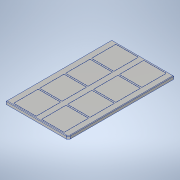
# Autodesk Inventor part: Assembly Plate
Saved by Autodesk Inventor 2022 (Build 260153000, 153)
## iProperties
Created: 2021-01-11
Part Number: Assembly Plate
Material: Aluminum 6061
Document SubType Name: Modeling
Designer: caleb
Density: 2.7 g/cm^3
Appearance: Aluminum - Flat
Author: caleb
Autodesk Inventor part; units mm, degrees
ref_plane "YZ Plane" through (0, 0, 0) normal (1, 0, 0) x (0, 1, 0)
ref_plane "XZ Plane" through (0, 0, 0) normal (0, 1, 0) x (-1, 0, 0)
ref_plane "XY Plane" through (0, 0, 0) normal (0, 0, 1) x (1, 0, 0)
sketch "Sketch1" plane through (0, 0, 0) normal (0, 1, 0) x (-1, 0, 0)
  line L0 (-63.5, 107.95) -> (63.5, 107.95)
  line L1 (63.5, 107.95) -> (63.5, -107.95)
  line L2 (63.5, -107.95) -> (-63.5, -107.95)
  line L3 (-63.5, -107.95) -> (-63.5, 107.95)
  line L4 (-63.5, 107.95) -> (63.5, -107.95) construction
  line L5 (63.5, 107.95) -> (-63.5, -107.95) construction
  point P0 (0, 0)
  dimension "d0" = 127
  dimension "d1" = 215.9
  constraints: 12 end point, 2 midpoint, 2 parallel, 1 horizontal, 1 perpendicular
  measures "d0" distance of L1.end L2.end
  measures "d1" distance of L0.end L1.end
extrude "Extrusion1" add sketch "Sketch1" along normal blind 6.35
sketch "Sketch8" plane through (0, 6.35, 0) normal (0, 1, 0) x (1, 0, 0)
  line L0 (-50.5, 104.45) -> (-6.5, 104.45)
  line L1 (-5.5, 103.45) -> (-5.5, 55.45)
  line L2 (-6.5, 54.45) -> (-50.5, 54.45)
  line L3 (-51.5, 55.45) -> (-51.5, 103.45)
  line L4 (63.5, 107.95) -> (-63.5, 107.95) projected
  line L5 (-63.5, -107.95) -> (63.5, -107.95) projected
  line L6 (-63.5, 107.95) -> (-63.5, -107.95) projected
  line L7 (63.5, -107.95) -> (63.5, 107.95) projected
  arc A0 (-51.5, 55.45) -> (-50.5, 54.45) centre (-50.5, 55.45) ccw
  arc A1 (-6.5, 54.45) -> (-5.5, 55.45) centre (-6.5, 55.45) ccw
  arc A2 (-5.5, 103.45) -> (-6.5, 104.45) centre (-6.5, 103.45) ccw
  arc A3 (-50.5, 104.45) -> (-51.5, 103.45) centre (-50.5, 103.45) ccw
  line L8 (-50.5, 51.45) -> (-6.5, 51.45)
  arc A4 (-50.5, 51.45) -> (-51.5, 50.45) centre (-50.5, 50.45) ccw
  arc A5 (-5.5, 50.45) -> (-6.5, 51.45) centre (-6.5, 50.45) ccw
  line L9 (-51.5, 2.45) -> (-51.5, 50.45)
  line L10 (-5.5, 50.45) -> (-5.5, 2.45)
  line L11 (-6.5, 1.45) -> (-50.5, 1.45)
  arc A6 (-6.5, 1.45) -> (-5.5, 2.45) centre (-6.5, 2.45) ccw
  arc A7 (-51.5, 2.45) -> (-50.5, 1.45) centre (-50.5, 2.45) ccw
  line L12 (-50.5, -1.55) -> (-6.5, -1.55)
  arc A8 (-50.5, -1.55) -> (-51.5, -2.55) centre (-50.5, -2.55) ccw
  arc A9 (-5.5, -2.55) -> (-6.5, -1.55) centre (-6.5, -2.55) ccw
  line L13 (-51.5, -50.55) -> (-51.5, -2.55)
  line L14 (-5.5, -2.55) -> (-5.5, -50.55)
  line L15 (-6.5, -51.55) -> (-50.5, -51.55)
  arc A10 (-6.5, -51.55) -> (-5.5, -50.55) centre (-6.5, -50.55) ccw
  arc A11 (-51.5, -50.55) -> (-50.5, -51.55) centre (-50.5, -50.55) ccw
  line L16 (-50.5, -54.55) -> (-6.5, -54.55)
  arc A12 (-50.5, -54.55) -> (-51.5, -55.55) centre (-50.5, -55.55) ccw
  arc A13 (-5.5, -55.55) -> (-6.5, -54.55) centre (-6.5, -55.55) ccw
  line L17 (-51.5, -103.55) -> (-51.5, -55.55)
  line L18 (-5.5, -55.55) -> (-5.5, -103.55)
  line L19 (-6.5, -104.55) -> (-50.5, -104.55)
  arc A14 (-6.5, -104.55) -> (-5.5, -103.55) centre (-6.5, -103.55) ccw
  arc A15 (-51.5, -103.55) -> (-50.5, -104.55) centre (-50.5, -103.55) ccw
  line L20 (6.5, 104.45) -> (50.5, 104.45)
  arc A16 (6.5, 104.45) -> (5.5, 103.45) centre (6.5, 103.45) ccw
  arc A17 (51.5, 103.45) -> (50.5, 104.45) centre (50.5, 103.45) ccw
  line L21 (5.5, 55.45) -> (5.5, 103.45)
  line L22 (51.5, 103.45) -> (51.5, 55.45)
  line L23 (50.5, 54.45) -> (6.5, 54.45)
  arc A18 (50.5, 54.45) -> (51.5, 55.45) centre (50.5, 55.45) ccw
  arc A19 (5.5, 55.45) -> (6.5, 54.45) centre (6.5, 55.45) ccw
  line L24 (6.5, 51.45) -> (50.5, 51.45)
  arc A20 (6.5, 51.45) -> (5.5, 50.45) centre (6.5, 50.45) ccw
  arc A21 (51.5, 50.45) -> (50.5, 51.45) centre (50.5, 50.45) ccw
  line L25 (5.5, 2.45) -> (5.5, 50.45)
  line L26 (51.5, 50.45) -> (51.5, 2.45)
  line L27 (50.5, 1.45) -> (6.5, 1.45)
  arc A22 (50.5, 1.45) -> (51.5, 2.45) centre (50.5, 2.45) ccw
  arc A23 (5.5, 2.45) -> (6.5, 1.45) centre (6.5, 2.45) ccw
  line L28 (6.5, -1.55) -> (50.5, -1.55)
  arc A24 (6.5, -1.55) -> (5.5, -2.55) centre (6.5, -2.55) ccw
  arc A25 (51.5, -2.55) -> (50.5, -1.55) centre (50.5, -2.55) ccw
  line L29 (5.5, -50.55) -> (5.5, -2.55)
  line L30 (51.5, -2.55) -> (51.5, -50.55)
  line L31 (50.5, -51.55) -> (6.5, -51.55)
  arc A26 (50.5, -51.55) -> (51.5, -50.55) centre (50.5, -50.55) ccw
  arc A27 (5.5, -50.55) -> (6.5, -51.55) centre (6.5, -50.55) ccw
  line L32 (6.5, -54.55) -> (50.5, -54.55)
  arc A28 (6.5, -54.55) -> (5.5, -55.55) centre (6.5, -55.55) ccw
  arc A29 (51.5, -55.55) -> (50.5, -54.55) centre (50.5, -55.55) ccw
  line L33 (5.5, -103.55) -> (5.5, -55.55)
  line L34 (51.5, -55.55) -> (51.5, -103.55)
  line L35 (50.5, -104.55) -> (6.5, -104.55)
  arc A30 (50.5, -104.55) -> (51.5, -103.55) centre (50.5, -103.55) ccw
  arc A31 (5.5, -103.55) -> (6.5, -104.55) centre (6.5, -103.55) ccw
  point P0 (0, 0)
  point P1 (-51.5, 104.45)
  point P2 (-5.5, 104.45)
  point P3 (-51.5, 54.45)
  point P4 (-51.5, 51.45)
  point P5 (-5.5, 51.45)
  point P6 (-51.5, 1.45)
  point P7 (-51.5, -1.55)
  point P8 (-5.5, -1.55)
  point P9 (-51.5, -51.55)
  point P10 (-51.5, -54.55)
  point P11 (-5.5, -54.55)
  point P12 (-51.5, -104.55)
  point P13 (5.5, 104.45)
  point P14 (51.5, 104.45)
  point P15 (5.5, 54.45)
  point P16 (5.5, 51.45)
  point P17 (51.5, 51.45)
  point P18 (5.5, 1.45)
  point P19 (5.5, -1.55)
  point P20 (51.5, -1.55)
  point P21 (5.5, -51.55)
  point P22 (5.5, -54.55)
  point P23 (51.5, -54.55)
  point P24 (5.5, -104.55)
  dimension "d92" = 46
  dimension "d93" = 50
  dimension "d102" = 3.5
  dimension "d104" = 12
  dimension "d106" = 1
  dimension "d109" = 53
  dimension "d112" = 57
  constraints: 64 end point, 64 point on circle, 48 point on line, 32 centre point, 8 tangent, 3 equal radius, 2 horizontal, 2 parallel, 1 collinear, 1 perpendicular, 1 vertical, 160 other
  measures "d92" distance of point (-51.5, 104.45) point (-5.5, 104.45)
  measures "d93" distance of point (-51.5, 54.45) point (-51.5, 104.45)
  measures "d102" distance between parallel lines of L4 L0
  measures "d104" distance between parallel lines of L6 L3
  measures "d106" radius of A0
  measures "d109" distance of point (-51.5, 104.45) point (-51.5, 51.45)
  measures "d112" distance of point (-51.5, 104.45) point (5.5, 104.45)
extrude "Extrusion7" cut sketch "Sketch8" against normal blind 0.2 contours L0 A2 L1 A1 L2 A0 L3 A3 | L8 A5 L10 A6 L11 A7 L9 A4 | L12 A9 L14 A10 L15 A11 L13 A8 | L16 A13 L18 A14 L19 A15 L17 A12 | L20 A17 L22 A18 L23 A19 L21 A16 | L24 A21 L26 A22 L27 A23 L25 A20 | L28 A25 L30 A26 L31 A27 L29 A24 | L32 A29 L34 A30 L35 A31 L33 A28
chamfer "Chamfer1" distance 4 angle 45 1 edges at (63.5, 3.175, 107.95)
chamfer "Chamfer2" distance 1 angle 45 4 edges at (63.5, 6.35, -2) (0, 6.35, -107.95) (-63.5, 6.35, 0) (-2, 6.35, 107.95)
chamfer "Chamfer3" distance 1 angle 45 1 edges at (61.5, 6.35, 105.95)
body "Solid1"
